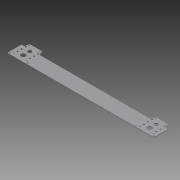
# Autodesk Inventor part: am-2952 AM14U2 Inside Sheet Mec Mod
Saved by Autodesk Inventor 2015 (Build 190159000, 159)
## iProperties
Created: 2015-01-10
Part Number: am-2952 AM14U2 Inside Sheet Mec Mod
Material: Generic
Document SubType Name: Modeling
Designer: whitaus15
Density: 1 g/cm^3
Appearance: Default
Author: whitaus15
Autodesk Inventor part; units mm, degrees
ref_plane "YZ Plane" through (0, 0, 0) normal (1, 0, 0) x (0, 1, 0)
ref_plane "XZ Plane" through (0, 0, 0) normal (0, 1, 0) x (-1, 0, 0)
ref_plane "Work Plane2" through (0, 130.175, -69.85) normal (0, 1, 0) x (1, 0, 0)
sketch "Sketch3" plane through (0, 130.175, -69.85) normal (0, 1, 0) x (1, 0, 0)
  line L0 (466.5934, -88.9) -> (346.2066, -88.9) projected
  arc A0 (343.457, -87.3125) -> (346.2066, -88.9) centre (346.2066, -85.725) ccw projected
  line L1 (334.2915, -71.4375) -> (343.457, -87.3125) projected
  line L2 (453.2877, 2.1413) -> (445.3167, 25.2907) projected
  arc A1 (445.3167, 25.2907) -> (442.3147, 27.432) centre (442.3147, 24.257) ccw projected
  line L3 (370.4853, 27.432) -> (442.3147, 27.432) projected
  arc A2 (370.4853, 27.432) -> (367.4833, 25.2907) centre (370.4853, 24.257) ccw projected
  line L4 (367.4833, 25.2907) -> (359.5123, 2.1413) projected
  arc A3 (356.5103, 0) -> (359.5123, 2.1413) centre (356.5103, 3.175) ccw projected
  line L5 (355.6, 0) -> (356.5103, 0) projected
  line L6 (355.6, 0) -> (0, 0) projected
  line L7 (0, 0) -> (0, -69.85) projected
  line L8 (0, -69.85) -> (330.2, -69.85) projected
  line L9 (330.2, -69.85) -> (331.5419, -69.85) projected
  arc A4 (334.2915, -71.4375) -> (331.5419, -69.85) centre (331.5419, -73.025) ccw projected
  line L10 (334.2915, -71.4375) -> (343.457, -87.3125) projected
  arc A5 (343.457, -87.3125) -> (346.2066, -88.9) centre (346.2066, -85.725) ccw projected
  line L11 (466.5934, -88.9) -> (346.2066, -88.9) projected
  arc A6 (466.5934, -88.9) -> (469.343, -87.3125) centre (466.5934, -85.725) ccw projected
  line L12 (469.343, -87.3125) -> (478.5085, -71.4375) projected
  arc A7 (481.2581, -69.85) -> (478.5085, -71.4375) centre (481.2581, -73.025) ccw projected
  line L13 (481.2581, -69.85) -> (482.6, -69.85) projected
  line L14 (482.6, -69.85) -> (812.8, -69.85) projected
  line L15 (812.8, -69.85) -> (812.8, 0) projected
  line L16 (812.8, 0) -> (457.2, 0) projected
  line L17 (456.2897, 0) -> (457.2, 0) projected
  arc A8 (453.2877, 2.1413) -> (456.2897, 0) centre (456.2897, 3.175) ccw projected
  circle A9 centre (619.3642, -13.4813) radius 2.667 projected
  circle A10 centre (193.4358, -13.4813) radius 2.667 projected
  circle A11 centre (193.4358, -60.1787) radius 2.667 projected
  arc A12 (666.4551, -57.5409) -> (666.4551, -62.8165) centre (666.0616, -60.1787) ccw projected
  arc A13 (666.4551, -62.8165) -> (666.4551, -57.5409) centre (666.8486, -60.1787) ccw projected
  arc A14 (146.3449, -16.1191) -> (146.3449, -10.8435) centre (146.7384, -13.4813) ccw projected
  arc A15 (146.3449, -10.8435) -> (146.3449, -16.1191) centre (145.9514, -13.4813) ccw projected
  arc A16 (146.3449, -62.8165) -> (146.3449, -57.5409) centre (146.7384, -60.1787) ccw projected
  arc A17 (146.3449, -57.5409) -> (146.3449, -62.8165) centre (145.9514, -60.1787) ccw projected
  arc A18 (666.4551, -10.8435) -> (666.4551, -16.1191) centre (666.0616, -13.4813) ccw projected
  arc A19 (666.4551, -16.1191) -> (666.4551, -10.8435) centre (666.8486, -13.4813) ccw projected
  circle A20 centre (170.0871, -36.83) radius 9.525 projected
  circle A21 centre (619.3642, -60.1787) radius 2.667 projected
  circle A22 centre (642.7129, -36.83) radius 9.525 projected
  circle A23 centre (122.6027, -36.83) radius 9.525 projected
  circle A24 centre (99.254, -60.1787) radius 2.667 projected
  circle A25 centre (99.254, -13.4813) radius 2.667 projected
  circle A26 centre (713.546, -13.4813) radius 2.667 projected
  circle A27 centre (713.546, -60.1787) radius 2.667 projected
  circle A28 centre (690.1973, -36.83) radius 9.525 projected
  circle A29 centre (461.9625, -82.7405) radius 3.4036 projected
  circle A30 centre (350.8375, -82.7405) radius 3.4036 projected
  circle A31 centre (711.2, -3.175) radius 1.27 projected
  circle A32 centre (711.2, -66.675) radius 1.27 projected
  circle A33 centre (762, -66.675) radius 1.27 projected
  circle A34 centre (762, -3.175) radius 1.27 projected
  circle A35 centre (50.8, -66.675) radius 1.27 projected
  circle A36 centre (50.8, -3.175) radius 1.27 projected
  circle A37 centre (101.6, -3.175) radius 1.27 projected
  circle A38 centre (101.6, -66.675) radius 1.27 projected
  circle A39 centre (806.45, -30.353) radius 3.3528 projected
  circle A40 centre (6.35, -30.353) radius 3.3528 projected
  circle A41 centre (787.4, -8.128) radius 3.3528 projected
  circle A42 centre (685.8, -8.128) radius 3.3528 projected
  circle A43 centre (584.2, -8.128) radius 3.3528 projected
  circle A44 centre (533.4, -8.128) radius 3.3528 projected
  circle A45 centre (482.6, -8.128) radius 3.3528 projected
  circle A46 centre (25.4, -8.128) radius 3.3528 projected
  circle A47 centre (127, -8.128) radius 3.3528 projected
  circle A48 centre (228.6, -8.128) radius 3.3528 projected
  circle A49 centre (279.4, -8.128) radius 3.3528 projected
  circle A50 centre (330.2, -8.128) radius 3.3528 projected
  circle A51 centre (450.8881, -70.8889) radius 2.032 projected
  circle A52 centre (361.9119, -70.8889) radius 2.032 projected
  circle A53 centre (367.7539, -70.8889) radius 2.54 projected
  circle A54 centre (445.0461, -70.8889) radius 2.54 projected
  circle A55 centre (368.808, 18.0035) radius 2.032 projected
  circle A56 centre (443.992, 18.0035) radius 2.032 projected
  circle A57 centre (374.65, 18.0035) radius 2.54 projected
  circle A58 centre (438.15, 18.0035) radius 2.54 projected
  circle A59 centre (367.6757, 1.016) radius 4.7625 projected
  circle A60 centre (367.6757, -49.784) radius 4.7625 projected
  circle A61 centre (445.1243, -49.784) radius 4.7625 projected
  circle A62 centre (445.1243, 1.016) radius 4.7625 projected
  circle A63 centre (367.6757, -24.384) radius 4.7625 projected
  circle A64 centre (445.1243, -24.384) radius 4.7625 projected
  circle A65 centre (406.4, -11.8872) radius 11.1125 projected
  circle A66 centre (641.35, -55.118) radius 3.3528 projected
  circle A67 centre (546.1, -55.118) radius 3.3528 projected
  circle A68 centre (266.7, -55.118) radius 3.3528 projected
  circle A69 centre (171.45, -55.118) radius 3.3528 projected
  circle A70 centre (513.9255, -52.3027) radius 3.3528 projected
  circle A71 centre (298.8745, -52.3027) radius 3.3528 projected
  circle A72 centre (628.9477, -50.8) radius 4.826 projected
  circle A73 centre (601.4385, -50.8) radius 4.826 projected
  circle A74 centre (568.9249, -50.8) radius 4.826 projected
  circle A75 centre (243.8751, -50.8) radius 4.826 projected
  circle A76 centre (211.3615, -50.8) radius 4.826 projected
  circle A77 centre (183.8523, -50.8) radius 4.826 projected
  circle A78 centre (678.9442, -49.022) radius 4.826 projected
  circle A79 centre (701.4504, -49.022) radius 4.826 projected
  circle A80 centre (726.4609, -49.022) radius 4.826 projected
  circle A81 centre (133.8558, -49.022) radius 4.826 projected
  circle A82 centre (111.3496, -49.022) radius 4.826 projected
  circle A83 centre (86.3391, -49.022) radius 4.826 projected
  circle A84 centre (406.4, -52.578) radius 14.2875 projected
  line L18 (826.5143, 100.4197) -> (706.1275, 100.4197)
  line L19 (813.2086, 191.4611) -> (805.2376, 214.6104)
  arc A85 (805.2376, 214.6104) -> (802.2356, 216.7517) centre (802.2356, 213.5767) ccw
  line L20 (730.4062, 216.7517) -> (802.2356, 216.7517)
  arc A86 (730.4062, 216.7517) -> (727.4042, 214.6104) centre (730.4062, 213.5767) ccw
  line L21 (727.4042, 214.6104) -> (719.4332, 191.4611)
  arc A87 (716.4312, 189.3197) -> (719.4332, 191.4611) centre (716.4312, 192.4947) ccw
  line L22 (715.5209, 189.3197) -> (716.4312, 189.3197)
  line L23 (826.5143, 100.4197) -> (706.1275, 100.4197)
  arc A88 (826.5143, 100.4197) -> (829.2639, 102.0072) centre (826.5143, 103.5947) ccw
  line L24 (816.2106, 189.3197) -> (817.1209, 189.3197)
  arc A89 (813.2086, 191.4611) -> (816.2106, 189.3197) centre (816.2106, 192.4947) ccw
  circle A90 centre (821.8834, 106.5792) radius 3.4036
  circle A91 centre (710.7584, 106.5792) radius 3.4036
  circle A92 centre (810.809, 118.4309) radius 2.032
  circle A93 centre (721.8328, 118.4309) radius 2.032
  circle A94 centre (727.6748, 118.4309) radius 2.54
  circle A95 centre (804.967, 118.4309) radius 2.54
  circle A96 centre (728.7289, 207.3233) radius 2.032
  circle A97 centre (803.9129, 207.3233) radius 2.032
  circle A98 centre (734.5709, 207.3233) radius 2.54
  circle A99 centre (798.0709, 207.3233) radius 2.54
  circle A100 centre (727.5966, 190.3357) radius 4.7625
  circle A101 centre (727.5966, 139.5357) radius 4.7625
  circle A102 centre (805.0452, 139.5357) radius 4.7625
  circle A103 centre (805.0452, 190.3357) radius 4.7625
  circle A104 centre (727.5966, 164.9357) radius 4.7625
  circle A105 centre (805.0452, 164.9357) radius 4.7625
  circle A106 centre (766.3209, 177.4325) radius 11.1125
  circle A107 centre (766.3209, 136.7417) radius 14.2875
  line L25 (817.1209, 189.3197) -> (829.2639, 189.3197)
  line L26 (829.2639, 189.3197) -> (829.2639, 102.0072)
  line L27 (715.5209, 189.3197) -> (706.1275, 189.3197)
  line L28 (706.1275, 100.4197) -> (372.0639, 100.4197)
  line L29 (706.1275, 189.3197) -> (372.0639, 189.3197)
  line L30 (372.0639, 189.3197) -> (372.0639, 100.4197)
  circle A108 centre (-60.9174, 139.5357) radius 4.7625
  circle A109 centre (-60.8392, 118.4309) radius 2.54
  circle A110 centre (-66.6812, 118.4309) radius 2.032
  circle A111 centre (-77.7556, 106.5792) radius 3.4036
  arc A112 (-85.1361, 102.0072) -> (-82.3864, 100.4197) centre (-82.3864, 103.5947) ccw
  circle A113 centre (-60.9174, 164.9357) radius 4.7625
  line L31 (-72.0828, 189.3197) -> (-72.9931, 189.3197)
  arc A114 (-72.0828, 189.3197) -> (-69.0807, 191.4611) centre (-72.0828, 192.4947) ccw
  circle A115 centre (-60.9174, 190.3357) radius 4.7625
  circle A116 centre (-59.7851, 207.3233) radius 2.032
  circle A117 centre (-53.9431, 207.3233) radius 2.54
  arc A118 (16.7237, 214.6104) -> (13.7216, 216.7517) centre (13.7216, 213.5767) ccw
  line L32 (16.7237, 214.6104) -> (24.6946, 191.4611)
  arc A119 (24.6946, 191.4611) -> (27.6966, 189.3197) centre (27.6966, 192.4947) ccw
  line L33 (28.6069, 189.3197) -> (27.6966, 189.3197)
  circle A120 centre (16.5312, 190.3357) radius 4.7625
  circle A121 centre (9.5569, 207.3233) radius 2.54
  circle A122 centre (15.3989, 207.3233) radius 2.032
  line L34 (-82.3864, 100.4197) -> (38.0003, 100.4197)
  circle A123 centre (33.3694, 106.5792) radius 3.4036
  circle A124 centre (22.295, 118.4309) radius 2.032
  circle A125 centre (16.453, 118.4309) radius 2.54
  circle A126 centre (16.5312, 139.5357) radius 4.7625
  circle A127 centre (16.5312, 164.9357) radius 4.7625
  circle A128 centre (-22.1931, 136.7417) radius 14.2875
  circle A129 centre (-22.1931, 177.4325) radius 11.1125
  line L35 (13.7216, 216.7517) -> (-58.1078, 216.7517)
  arc A130 (-58.1078, 216.7517) -> (-61.1098, 214.6104) centre (-58.1078, 213.5767) ccw
  line L36 (-69.0807, 191.4611) -> (-61.1098, 214.6104)
  line L37 (-82.3864, 100.4197) -> (38.0003, 100.4197)
  line L38 (-72.9931, 189.3197) -> (-85.1361, 189.3197)
  line L39 (-85.1361, 189.3197) -> (-85.1361, 102.0072)
  line L40 (28.6069, 189.3197) -> (38.0003, 189.3197)
  line L41 (38.0003, 100.4197) -> (372.0639, 100.4197)
  line L42 (38.0003, 189.3197) -> (372.0639, 189.3197)
  dimension "d7" = 123.1364
  dimension "d8" = 457.2
  constraints: 50 end point, 46 centre point, 40 symmetric about line, 20 point on circle, 3 horizontal, 2 perpendicular, 2 point on line, 23 other
  measures "d7" distance from line of L18.end L26
  measures "d8" distance from line of L28.end L26
extrude "Extrusion3" add sketch "Sketch3" along normal blind 3.175 contours L18 L28 L30 L29 L27 L22 A87 L21 A86 L20 A85 L19 A89 L24 L25 L26 A88 | L41 L34 A112 L39 L38 L31 A114 L36 A130 L35 A118 L32 A119 L33 L40 L42 L30
